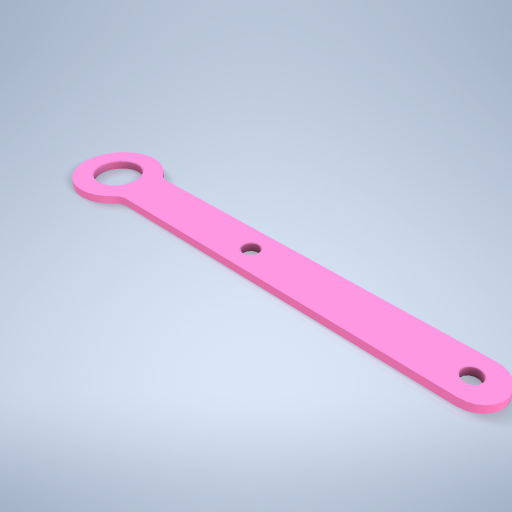
# Autodesk Inventor part: pleuel
Saved by Autodesk Inventor 2024.2 (Build 282272000, 272)
## iProperties
Created: 2024-04-18
Part Number: pleuel
Material: Edelstahl, 440C
Document SubType Name: Modeling
Designer: Fabri
Density: 7.75 g/cm^3
Appearance: Pink
Author: Fabri
Autodesk Inventor part; units mm, degrees
ref_plane "YZ Plane" through (0, 0, 0) normal (1, 0, 0) x (0, 1, 0)
ref_plane "XZ Plane" through (0, 0, 0) normal (0, 1, 0) x (-1, 0, 0)
ref_plane "XY Plane" through (0, 0, 0) normal (0, 0, 1) x (1, 0, 0)
sketch "Skizze1" plane through (0, 0, 0) normal (0, 0, 1) x (1, 0, 0)
  line L0 (0, 0) -> (38.7995, 0) construction
  arc A0 (4.6098, 3) -> (4.6098, -3) centre (0, 0) ccw
  circle A1 centre (0, 0) radius 3
  line L1 (4.6098, 3) -> (4.6098, -3)
  line L2 (4.6098, 3) -> (50, 3)
  line L3 (53, 0) -> (53, 0)
  line L4 (50, -3) -> (4.6098, -3)
  arc A2 (53, 0) -> (50, 3) centre (50, 0) ccw
  arc A3 (50, -3) -> (53, 0) centre (50, 0) ccw
  point P0 (53, 0)
  dimension "d1" = 6
  dimension "d4" = 6
  dimension "d5" = 5.5
  dimension "d6" = 3
  dimension "d7" = 50
  constraints: 10 end point, 6 point on circle, 4 centre point, 4 tangent, 2 coincident, 2 horizontal, 2 perpendicular, 1 concentric, 1 symmetric about line
  measures "d1" diameter of A1
  measures "d4" distance of L1.end L1.start
  measures "d5" radius of A0
  measures "d6" radius of A2
  measures "d7" distance of A3.centre L0.start
extrude "Extrusion1" add sketch "Skizze1" along normal blind 1
fillet "Rundung1" radius 2 2 edges at (4.6098, 3, 0.5) (4.6098, -3, 0.5)
sketch "Skizze3" plane through (0, 0, 0) normal (0, 0, -1) x (-1, 0, 0)
  point P0 (0, 0)
  point P1 (-49.5, 0)
  dimension "d26" = 49.5
  constraints: 1 horizontal alignment
  measures "d26" distance of point (0, 0) point (-49.5, 0)
hole "Bohrung2" at (49.5, 0, 0) direction (0, 0, 1) diameter 2.2 depth 1
sketch "Skizze2" plane through (0, 0, 1) normal (0, 0, 1) x (1, 0, 0)
  point P0 (0, 0)
  point P1 (23, 0)
  dimension "d18" = 23
  constraints: 1 horizontal alignment
  measures "d18" distance of point (23, 0) point (0, 0)
hole "Bohrung1" at (23, 0, 1) direction (0, 0, -1) diameter 2.2 depth 1
